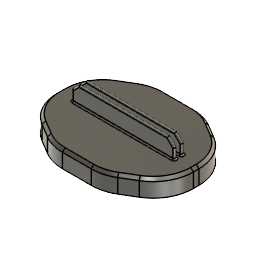
Undergrad Project (Autodesk Fusion 360 design; units mm, degrees)
part number: 2025-11-23-22-00-11-729
Autodesk Fusion 360 part; units mm, degrees
sketch "leg" plane through (0, 0, 0) normal (0, 0, 1) x (1, 0, 0)
  line L0 (-250.3486, 82.3044) -> (-199.5486, 82.3044)
  line L1 (-199.5486, 82.3044) -> (-199.5486, -19.2956)
  line L2 (-199.5486, -19.2956) -> (-250.3486, -19.2956)
  line L3 (-250.3486, -19.2956) -> (-250.3486, 82.3044)
  dimension "d9" = 50.8
  dimension "d10" = 101.6
  constraint horizontal L0
  constraint vertical L1
  constraint horizontal L2
  constraint vertical L3
  measures "d9" distance of L0.start L0.end
  measures "d10" distance of L0.start L2.end
extrude "Extrude1" add sketch "leg" along normal blind 38.1 makes body 1
move_body "Move2" bodies 1 to x (1, 0, 0) y (0, 1, 0) z (0, 0, 1) at (-290, 0, 0)
sketch "top of left leg and cross" plane through (0, 0, 38.1) normal (0, 0, 1) x (-1, 0, 0)
  line L0 (540.3486, 19.2956) -> (489.5486, 19.2956)
  line L1 (489.5486, 19.2956) -> (489.5486, -82.3044)
  line L2 (489.5486, -82.3044) -> (540.3486, -82.3044)
  line L3 (540.3486, -82.3044) -> (540.3486, 19.2956)
  line L4 (540.3486, -82.3044) -> (489.5486, 19.2956) construction
  line L5 (489.5486, -82.3044) -> (540.3486, 19.2956) construction
  line L6 (514.9486, -31.5044) -> (514.5014, -32.3989) construction
  line L7 (514.9486, -31.5044) -> (514.9486, -44.2044) construction
  line L8 (514.9486, -31.5044) -> (514.9486, -18.8044) construction
  line L9 (514.9486, -44.2044) -> (-73.1058, -44.2044)
  line L10 (-73.1058, -44.2044) -> (-73.1058, -18.8044)
  line L11 (-73.1058, -18.8044) -> (514.9486, -18.8044)
  line L12 (514.9486, -18.8044) -> (514.9486, -44.2044)
  dimension "d16" = 12.7
  dimension "d17" = 12.7
  dimension "d18" = 588.0544
  dimension "d19" = 25.4
  constraint coincident L2.end L3.start
  constraint coincident L0.end L1.start
  constraint coincident L1.end L2.start
  constraint coincident L0.start L3.end
  constraint midpoint L4 L6.start
  constraint vertical L7
  constraint vertical L8
  constraint horizontal L9
  constraint vertical L10
  constraint horizontal L11
  constraint vertical L12
  measures "d16" distance of L6.start L7.end
  measures "d17" distance of L6.start L8.end
  measures "d18" distance of L7.end L9.end
  measures "d19" distance of L7.end L8.end
copy_body "CopyPasteBodies2" bodies 1 makes body 2
move_body "Move4" bodies 2 to x (1, 0, 0) y (0, 1, 0) z (0, 0, 1) at (587.6544, 0, 0)
sketch "top of right leg" plane through (0, 0, 38.1) normal (0, 0, 1) x (-1, 0, 0)
  line L0 (-47.3058, 19.2956) -> (-98.1058, 19.2956)
  line L1 (-98.1058, 19.2956) -> (-98.1058, -82.3044)
  line L2 (-98.1058, -82.3044) -> (-47.3058, -82.3044)
  line L3 (-47.3058, -82.3044) -> (-47.3058, 19.2956)
  line L4 (-47.3058, -82.3044) -> (-98.1058, 19.2956) construction
  line L5 (-98.1058, -82.3044) -> (-47.3058, 19.2956) construction
  line L6 (-72.7058, -31.5044) -> (-72.7058, -44.2044) construction
  line L7 (-72.7058, -31.5044) -> (-72.7058, -18.8044) construction
  dimension "d22" = 12.7
  dimension "d23" = 12.7
  constraint coincident L2.end L3.start
  constraint coincident L0.end L1.start
  constraint coincident L1.end L2.start
  constraint coincident L0.start L3.end
  constraint midpoint L5 L6.start
  constraint parallel L3 L6
  constraint parallel L6 L7
  measures "d22" distance of L6.start L6.end
  measures "d23" distance of L6.start L7.end
extrude "Extrude2" add sketch "top of left leg and cross" along normal blind 12.7 contours L1 L9 L11 L12 | L1 L9 L10 L11 bodies 1 2
move_body "Move5" bodies 1 to x (1, 0, 0) y (0, 1, 0) z (0, 0, 1) at (0.4, 0, 0)
extrude "Extrude3" add 1 faces at (-514.5486, 27.2711, 42.3333) along direction (-1, 0, 0) blind 2 on bodies 1 bodies 1
extrude "Extrude4" add 1 faces at (73.5058, 35.7378, 42.3333) along direction (1, 0, 0) blind 2 on bodies 1 bodies 1
sketch "Sketch8" plane through (0, 0, 50.8) normal (0, 0, 1) x (-1, 0, 0)
  line L0 (516.5486, -18.8044) -> (-75.5058, -18.8044)
  line L1 (-75.5058, -18.8044) -> (-75.5058, -44.2044)
  line L2 (-75.5058, -44.2044) -> (516.5486, -44.2044)
  line L3 (516.5486, -44.2044) -> (516.5486, -18.8044)
  line L4 (-75.5058, -44.2044) -> (516.5486, -18.8044) construction
  line L5 (516.5486, -44.2044) -> (-75.5058, -18.8044) construction
  line L6 (220.5214, -31.5044) -> (220.5214, -18.8044) construction
  line L7 (220.5214, -31.5044) -> (220.5214, -44.2044) construction
  line L8 (516.5486, -44.2044) -> (514.5486, -44.2044) construction
  line L9 (514.5486, -44.2044) -> (514.5486, -18.8044) construction
  line L10 (514.5486, -18.8044) -> (516.5486, -18.8044) construction
  line L11 (516.5486, -18.8044) -> (516.5486, -44.2044) construction
  line L12 (-75.5058, -44.2044) -> (-73.5058, -44.2044) construction
  line L13 (-73.5058, -44.2044) -> (-73.5058, -18.8044) construction
  line L14 (-73.5058, -18.8044) -> (-75.5058, -18.8044) construction
  line L15 (-75.5058, -18.8044) -> (-75.5058, -44.2044) construction
  line L16 (-75.5058, -31.5044) -> (-70.5058, -31.5044) construction
  line L17 (-70.5058, -31.5044) -> (-70.5058, -31.8544) construction
  line L18 (-70.5058, -31.5044) -> (-70.5058, -31.1544) construction
  line L19 (-70.5058, -31.8544) -> (-73.5058, -31.8544) construction
  line L20 (-70.5058, -31.1544) -> (-73.5058, -31.1544) construction
  line L21 (-70.5058, -31.8544) -> (514.5486, -31.8544) construction
  line L22 (514.5486, -31.5044) -> (509.5486, -31.5044) construction
  line L23 (509.5486, -31.5044) -> (509.5486, -31.8544) construction
  line L24 (509.5486, -31.5044) -> (509.5486, -31.1544) construction
  line L25 (-70.5058, -31.1544) -> (514.5486, -31.1544) construction
  dimension "d32" = 2
  dimension "d33" = 25.4
  dimension "d34" = 2
  dimension "d35" = 25.4
  dimension "d36" = 5
  dimension "d37" = 0.35
  dimension "d38" = 0.35
  dimension "d39" = 5
  dimension "d40" = 0.35
  dimension "d41" = 0.35
  constraint coincident L1.end L2.start
  constraint coincident L0.start L3.end
  constraint coincident L2.end L3.start
  constraint coincident L0.end L1.start
  constraint midpoint L4 L6.start
  constraint midpoint L0 L6.end
  constraint midpoint L2 L7.end
  constraint horizontal L8
  constraint vertical L9
  constraint horizontal L10
  constraint vertical L11
  constraint horizontal L12
  constraint vertical L13
  constraint horizontal L14
  constraint vertical L15
  constraint midpoint L15 L16.start
  constraint perpendicular L15 L16
  constraint perpendicular L16 L17
  constraint perpendicular L16 L18
  constraint coincident L13 L19.end
  constraint perpendicular L13 L19
  constraint coincident L13 L20.end
  constraint perpendicular L13 L20
  constraint coincident L9 L21.end
  constraint perpendicular L9 L21
  constraint midpoint L9 L22.start
  constraint perpendicular L9 L22
  constraint perpendicular L22 L23
  constraint perpendicular L22 L24
  constraint coincident L9 L25.end
  constraint perpendicular L9 L25
  measures "d32" distance of L2.end L8.end
  measures "d33" distance of L2.end L0.start
  measures "d34" distance of L1.end L12.end
  measures "d35" distance of L1.end L0.end
  measures "d36" distance of L16.start L16.end
  measures "d37" distance of L16.end L17.end
  measures "d38" distance of L16.end L18.end
  measures "d39" distance of L22.start L22.end
  measures "d40" distance of L22.end L23.end
  measures "d41" distance of L22.end L24.end
sketch "base" plane through (0, 0, 0) normal (0, 0, 1) x (1, 0, 0)
  line L0 (0, 0) -> (50.8, 0) construction
  line L1 (0, 0) -> (-50.8, 0) construction
  line L2 (0, 0) -> (0, 38.1) construction
  line L3 (0, 0) -> (0, -38.1) construction
  line L4 (-50.8, 0) -> (-50.8, 19.05)
  line L5 (-50.8, 0) -> (-50.8, -19.05)
  line L6 (50.8, 0) -> (50.8, 19.05)
  line L7 (50.8, 0) -> (50.8, -19.05)
  line L8 (0, -38.1) -> (19.05, -38.1)
  line L9 (0, -38.1) -> (-19.05, -38.1)
  line L10 (0, 38.1) -> (-19.05, 38.1)
  line L11 (0, 38.1) -> (19.05, 38.1)
  line L12 (-50.8, -19.05) -> (-19.05, -38.1)
  line L13 (19.05, -38.1) -> (50.8, -19.05)
  line L14 (50.8, 19.05) -> (19.05, 38.1)
  line L15 (-19.05, 38.1) -> (-50.8, 19.05)
  dimension "d42" = 50.8
  dimension "d43" = 50.8
  dimension "d44" = 38.1
  dimension "d45" = 38.1
  dimension "d46" = 19.05
  dimension "d47" = 19.05
  dimension "d48" = 19.05
  dimension "d49" = 19.05
  dimension "d50" = 19.05
  dimension "d51" = 19.05
  dimension "d52" = 19.05
  dimension "d53" = 19.05
  constraint coincident L0.start L1.start
  constraint horizontal L0
  constraint parallel L0 L1
  constraint perpendicular L0 L2
  constraint perpendicular L0 L3
  constraint perpendicular L1 L4
  constraint perpendicular L1 L5
  constraint perpendicular L0 L6
  constraint perpendicular L0 L7
  constraint perpendicular L3 L8
  constraint perpendicular L3 L9
  constraint perpendicular L2 L10
  constraint perpendicular L2 L11
  measures "d42" distance of L0.start L0.end
  measures "d43" distance of L0.start L1.end
  measures "d44" distance of L0.start L2.end
  measures "d45" distance of L0.start L3.end
  measures "d46" distance of L1.end L4.end
  measures "d47" distance of L1.end L5.end
  measures "d48" distance of L0.end L6.end
  measures "d49" distance of L0.end L7.end
  measures "d50" distance of L3.end L8.end
  measures "d51" distance of L3.end L9.end
  measures "d52" distance of L2.end L10.end
  measures "d53" distance of L2.end L11.end
extrude "Extrude5" add sketch "base" along normal blind 12.7 separate body makes body 3
sketch "rail" plane through (0, 0, 12.7) normal (0, 0, 1) x (-1, 0, 0)
  line L0 (-19.05, -38.1) -> (19.05, -38.1)
  line L1 (19.05, -38.1) -> (50.8, -19.05)
  line L2 (50.8, -19.05) -> (50.8, 19.05)
  line L3 (50.8, 19.05) -> (19.05, 38.1)
  line L4 (19.05, 38.1) -> (-19.05, 38.1)
  line L5 (-19.05, 38.1) -> (-50.8, 19.05)
  line L6 (-50.8, 19.05) -> (-50.8, -19.05)
  line L7 (-50.8, -19.05) -> (-19.05, -38.1)
  line L8 (0, 0) -> (0, -38.1) construction
  line L9 (0, 0) -> (-50.8, 0) construction
  line L10 (0, 0) -> (50.8, 0) construction
  line L11 (0, 0) -> (0, 38.1) construction
  line L12 (-38.1, -3.7) -> (38.1, -3.7)
  line L13 (38.1, -3.7) -> (38.1, 3.7)
  line L14 (38.1, 3.7) -> (-38.1, 3.7)
  line L15 (-38.1, 3.7) -> (-38.1, -3.7)
  line L16 (-38.1, -3.7) -> (38.1, 3.7) construction
  line L17 (38.1, -3.7) -> (-38.1, 3.7) construction
  line L18 (-38.1, -1.7) -> (38.1, -1.7)
  line L19 (38.1, -1.7) -> (38.1, 1.7)
  line L20 (38.1, 1.7) -> (-38.1, 1.7)
  line L21 (-38.1, 1.7) -> (-38.1, -1.7)
  line L22 (-38.1, -1.7) -> (38.1, 1.7) construction
  line L23 (38.1, -1.7) -> (-38.1, 1.7) construction
  dimension "d56" = 76.2
  dimension "d57" = 7.4
  dimension "d58" = 76.2
  dimension "d59" = 3.4
  constraint coincident L8.start L9.start
  constraint midpoint L0 L8.end
  constraint midpoint L6 L9.end
  constraint midpoint L2 L10.end
  constraint midpoint L4 L11.end
  constraint horizontal L12
  constraint perpendicular L12 L13
  constraint parallel L12 L14
  constraint parallel L13 L15
  constraint coincident L16 L8.start
  constraint coincident L17 L8.start
  constraint horizontal L18
  constraint perpendicular L18 L19
  constraint parallel L18 L20
  constraint parallel L19 L21
  constraint coincident L22 L8.start
  constraint coincident L23 L8.start
  measures "d56" distance of L13.end L14.end
  measures "d57" distance of L12.end L13.end
  measures "d58" distance of L19.end L20.end
  measures "d59" distance of L18.end L19.end
extrude "Extrude6" add sketch "rail" along normal blind 12.7 contours L12 L13 L15 L18 | L13 L14 L15 L20 bodies 3
fillet "Fillet1" radius 30 8 edges at (19.05, 38.1, 6.35) (-19.05, 38.1, 6.35) (50.8, 19.05, 6.35) (50.8, -19.05, 6.35) (19.05, -38.1, 6.35) (-19.05, -38.1, 6.35) (-50.8, -19.05, 6.35) (-50.8, 19.05, 6.35) on bodies 3
chamfer "Chamfer1" distance 2 angle 45 16 edges at (-31.2051, -30.8069, 12.7) (-18.7485, -37.0114, 12.7) (0, -38.1, 12.7) (18.7485, -37.0114, 12.7) (31.2051, -30.8069, 12.7) (46.906, -16.8453, 12.7) (50.8, 0, 12.7) (46.906, 16.8453, 12.7) (31.2051, 30.8069, 12.7) (18.7485, 37.0114, 12.7) (0, 38.1, 12.7) (-18.7485, 37.0114, 12.7) (-31.2051, 30.8069, 12.7) (-46.906, 16.8453, 12.7) (-50.8, 0, 12.7) (-46.906, -16.8453, 12.7) on bodies 3
chamfer "Chamfer2" distance 5 angle 45 4 edges at (38.1, -2.7, 25.4) (38.1, 2.7, 25.4) (-38.1, -2.7, 25.4) (-38.1, 2.7, 25.4) on bodies 3
fillet "Fillet2" radius 1 20 edges at (0, -3.7, 25.4) (0, -1.7, 25.4) (35.6, -3.7, 22.9) (35.6, -1.7, 22.9) (38.1, -3.7, 16.55) (38.1, -1.7, 16.55) (35.6, 1.7, 22.9) (38.1, 1.7, 16.55) (38.1, 3.7, 16.55) (35.6, 3.7, 22.9) (0, 3.7, 25.4) (0, 1.7, 25.4) (-35.6, -3.7, 22.9) (-35.6, -1.7, 22.9) (-38.1, -3.7, 16.55) (-38.1, -1.7, 16.55) (-38.1, 1.7, 16.55) (-38.1, 3.7, 16.55) (-35.6, 3.7, 22.9) (-35.6, 1.7, 22.9) on bodies 3
fillet "Fillet3" radius 1 8 edges at (-38.1, -2.7, 12.7) (0, -1.7, 12.7) (38.1, -2.7, 12.7) (0, -3.7, 12.7) (38.1, 2.7, 12.7) (0, 1.7, 12.7) (-38.1, 2.7, 12.7) (0, 3.7, 12.7) on bodies 3
hidden bodies 1
equation "legLength = 4 in"
equation "legWidth = 2 in"
equation "legHeight = 1.5 in"
equation "insertLength = 23.136 in"
equation "insertHeight = 3.867 in"
equation "insertWidth = 3 mm"
equation "d9 = legWidth"
equation "d10 = legLength"
equation "d11 = legHeight"
equation "d18 = insertLength + 0.4 mm"
equation "d42 = baseSize"
equation "d43 = baseSize"
equation "d44 = baseSize * 0.75"
equation "d45 = baseSize * 0.75"
equation "d57 = insertWidth + 4.4 mm"
equation "d59 = insertWidth + 0.4 mm"
equation "baseSize = 2 in"
named bodies: "leg1", "leg1 (1)", "leg2", "stand"
